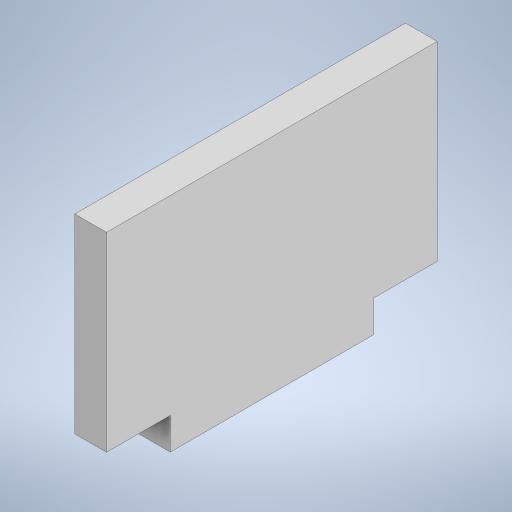
# Autodesk Inventor part: servo long side
Saved by Autodesk Inventor 2023 (Build 270158000, 158)
## iProperties
Created: 2023-10-15
Part Number: servo long side
Material: Generic
Document SubType Name: Modeling
Designer: Nate
Density: 1 g/cm^3
Appearance: Default
Author: Nate
Autodesk Inventor part; units mm, degrees
ref_plane "YZ Plane" through (0, 0, 0) normal (1, 0, 0) x (0, 1, 0)
ref_plane "XZ Plane" through (0, 0, 0) normal (0, 1, 0) x (-1, 0, 0)
ref_plane "XY Plane" through (0, 0, 0) normal (0, 0, 1) x (1, 0, 0)
sketch "Sketch1" plane through (0, 0, 0) normal (0, 0, 1) x (1, 0, 0)
  line L0 (0, 0) -> (-6.35, 0)
  line L1 (-6.35, 0) -> (-6.35, 40.64)
  line L2 (-6.35, 40.64) -> (0, 40.64)
  line L3 (0, 40.64) -> (0, 0)
  line L4 (-44.45, -12.7508) -> (-6.35, -12.7508)
  line L5 (-6.35, -12.7508) -> (-6.35, 53.3908)
  line L6 (-6.35, 53.3908) -> (-44.45, 53.3908)
  line L7 (-44.45, 53.3908) -> (-44.45, -12.7508)
  point P0 (-25.4, 53.3908)
  point P1 (-25.4, -12.7508)
  dimension "d0" = 6.35
  dimension "d1" = 40.64
  dimension "d2" = 66.1416
  dimension "d3" = 12.7508
  dimension "d5" = 38.1
  dimension "d6" = 0
  constraints: 16 end point, 4 parallel, 2 horizontal, 2 midpoint, 2 perpendicular
  measures "d0" distance of L1.end L2.end
  measures "d1" distance of L0.end L1.end
  measures "d2" distance of point (-25.4, 53.391) point (-25.4, -12.751)
  measures "d3" distance between parallel lines of L0 L4
  measures "d5" distance between parallel lines of L7 L1
  measures "d6" distance between parallel lines of L1 L5
extrude "Extrusion1" add sketch "Sketch1" along normal blind 6.35
move or copy body "Move Body1" bodies to move or copy 1 copy no rotation origin (0, 0, 0) rotation axis (0, 0, 1) rotation angle -90 translate (-40.64, 40.64, 0)
move or copy body "Move Body2" bodies to move or copy 1 copy no rotation origin (0, 0, 0) rotation axis (0, -1, 0) rotation angle -90 translate (12.7508, 0, 12.7508)
move or copy body "Move Body3" bodies to move or copy 1 copy no translate (25.4, 0, 0)
body "Solid1"
